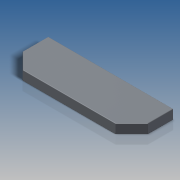
# Autodesk Inventor part: 11236-LtBluishGray
Saved by Autodesk Inventor 2016 SP2 (Build 200236200, 236)
## iProperties
Created: 2015-08-26
Part Number: 11236-LtBluishGray
Material: ABS Plastic
Document SubType Name: Modeling
Designer: D. Kohfeld
Density: 1.06 g/cm^3
Appearance: LtBluishGray
Mass: 0.250334 g
Surface Area: 3.79765 cm^2
Volume: 0.236164 cm^3
Author: D. Kohfeld
Autodesk Inventor part; units mm, degrees
ref_plane "YZ Plane" through (0, 0, 0) normal (1, 0, 0) x (0, 1, 0)
ref_plane "XZ Plane" through (0, 0, 0) normal (0, 1, 0) x (-1, 0, 0)
ref_plane "XY Plane" through (0, 0, 0) normal (0, 0, 1) x (1, 0, 0)
sketch "Sketch2" plane through (0, 0, 0) normal (0, 1, 0) x (-1, 0, 0)
  line L0 (-10.8, -4.4) -> (10.8, -4.4)
  line L1 (10.8, -4.4) -> (10.8, 0)
  line L2 (10.8, 0) -> (8, 2.8)
  line L3 (8, 2.8) -> (-8, 2.8)
  line L4 (-8, 2.8) -> (-10.8, 0)
  line L5 (-10.8, 0) -> (-10.8, -4.4)
  point P0 (0, 0)
  point P1 (0, -4.4)
  point P2 (0, 2.8)
  dimension "d0" = 16
  dimension "d1" = 21.6
  dimension "d2" = 7.2
  constraints: 12 end point, 2 equal length, 2 horizontal, 2 midpoint, 2 vertical, 2 vertical alignment, 1 horizontal alignment, 1 perpendicular
  measures "d0" distance of L2.end L3.end
  measures "d1" distance of L0.start L0.end
  measures "d2" distance between parallel lines of L3 L0
extrude "Extrusion1" add sketch "Sketch2" along normal mid plane 1.6
fillet "Fillet1" radius 0.1 12 edges at (-9.4, 0.8, 1.4) (-10.8, 0.8, -2.2) (0, 0.8, -4.4) (-8, 0, 2.8) (-10.8, 0, 0) (-10.8, 0, -4.4) (10.8, 0, -4.4) (10.8, 0.8, -2.2) (10.8, 0, 0) (9.4, 0.8, 1.4) (8, 0, 2.8) (0, 0.8, 2.8)
equation "\"d0\" = 2 * lu"
equation "\"d3\" = wall"
equation "\"lu\" = 8"
equation "\"wall\" = 1.6"
body "Solid1"
